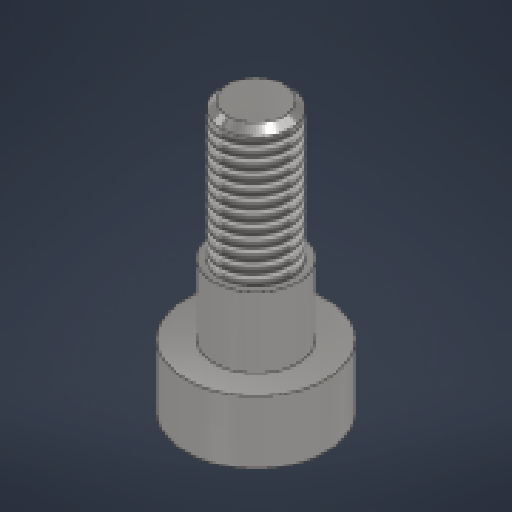
# Autodesk Inventor part: Ali_d5-M4
Saved by Autodesk Inventor 2024.3 (Build 283343000, 343)
## iProperties
Created: 2025-01-09
Part Number: Ali_d5-M4
Material: 스테인리스스틸
Document SubType Name: Modeling
Designer: ASUS
Density: 8 g/cm^3
Appearance: 반연마
Author: ASUS
Autodesk Inventor part; units mm, degrees
ref_plane "YZ Plane" through (0, 0, 0) normal (1, 0, 0) x (0, 1, 0)
ref_plane "XZ Plane" through (0, 0, 0) normal (0, 1, 0) x (-1, 0, 0)
ref_plane "XY Plane" through (0, 0, 0) normal (0, 0, 1) x (1, 0, 0)
sketch "스케치1" plane through (0, 0, 0) normal (0, 0, 1) x (1, 0, 0)
  line L0 (0, 0) -> (0, 20)
  line L1 (0, 0) -> (4.5, 0)
  line L2 (4.5, 0) -> (4.5, 3.5)
  line L3 (4.5, 3.5) -> (0, 3.5)
  line L4 (0, 3.5) -> (0, 0)
  line L5 (0, 3.5) -> (2.5, 3.5)
  line L6 (2.5, 3.5) -> (2.5, 8.5)
  line L7 (2.5, 8.5) -> (0, 8.5)
  line L8 (0, 8.5) -> (0, 3.5)
  line L9 (0, 8.5) -> (2, 8.5)
  line L10 (2, 8.5) -> (2, 16.5)
  line L11 (2, 16.5) -> (0, 16.5)
  line L12 (0, 16.5) -> (0, 8.5)
  point P0 (0, 16.5)
  point P1 (0, 3.5)
  point P2 (0, 8.5)
  dimension "d0" = 20
  dimension "d1" = 4.5
  dimension "d2" = 3.5
  dimension "d3" = 2.5
  dimension "d4" = 5
  dimension "d5" = 2
  dimension "d6" = 8
  constraints: 26 end point, 6 parallel, 4 perpendicular, 2 point on line, 1 vertical
  measures "d0" distance of L0.start L0.end
  measures "d1" distance of L0.start L1.end
  measures "d2" distance of L2.end L1.end
  measures "d3" distance of L3.end L5.end
  measures "d4" distance of L6.end L5.end
  measures "d5" distance of L7.end L9.end
  measures "d6" distance of L10.end L9.end
revolve "회전1" add sketch "스케치1" angle 360 about axis through (0, 16.5, 0) along (0, -1, 0)
chamfer "모따기1" distance 0.5 angle 45 1 edges at (-2, 16.5, 0)
thread "스레드2" size "M4x0.7" class "6g" standard "ANSI Metric M Profile" full length
